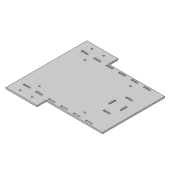
# Autodesk Inventor part: Chassis
Saved by Autodesk Inventor 2017 (Build 210142000, 142)
## iProperties
Created: 2019-06-10
Part Number: Chassis
Material: Generic
Document SubType Name: Modeling
Designer: markg
Density: 1 g/cm^3
Appearance: Default
Author: markg
Autodesk Inventor part; units mm, degrees
ref_plane "YZ Plane" through (0, 0, 0) normal (1, 0, 0) x (0, 1, 0)
ref_plane "XZ Plane" through (0, 0, 0) normal (0, 1, 0) x (-1, 0, 0)
ref_plane "XY Plane" through (0, 0, 0) normal (0, 0, 1) x (1, 0, 0)
sketch "Sketch1" plane through (0, 0, 0) normal (0, 1, 0) x (-1, 0, 0)
  line L0 (-88.9, 63.5) -> (88.9, 63.5)
  line L1 (88.9, 63.5) -> (88.9, -63.5)
  line L2 (88.9, -63.5) -> (-88.9, -63.5)
  line L3 (-88.9, -63.5) -> (-88.9, 63.5)
  line L4 (-88.9, 63.5) -> (88.9, -63.5) construction
  line L5 (88.9, 63.5) -> (-88.9, -63.5) construction
  point P0 (0, 0)
  dimension "d0" = 127
  dimension "d1" = 177.8
  constraints: 12 end point, 2 midpoint, 2 parallel, 1 horizontal, 1 perpendicular
  measures "d0" distance of L0.start L2.end
  measures "d1" distance of L2.end L1.end
extrude "Extrusion1" add sketch "Sketch1" along normal blind 2.921
sketch "Sketch2" plane through (0, 2.921, 0) normal (0, 1, 0) x (1, 0, 0)
  line L0 (-60.325, -50) -> (39.675, -50) construction
  line L1 (39.675, -50) -> (39.675, 50) construction
  line L2 (39.675, 50) -> (-60.325, 50) construction
  line L3 (-60.325, 50) -> (-60.325, -50) construction
  circle A0 centre (36.119, -46.444) radius 1.5875
  circle A1 centre (-56.769, -46.444) radius 1.5875
  circle A2 centre (-56.769, 46.444) radius 1.5875
  circle A3 centre (36.119, 46.444) radius 1.5875
  point P0 (0, 0)
  dimension "d8" = 100
  dimension "d9" = 100
  dimension "d10" = 50
  dimension "d11" = 60.325
  dimension "d12" = 3.175
  dimension "d13" = 3.175
  dimension "d14" = 3.175
  dimension "d15" = 3.175
  dimension "d16" = 3.556
  dimension "d17" = 3.556
  dimension "d18" = 3.556
  dimension "d19" = 3.556
  dimension "d20" = 3.556
  dimension "d21" = 3.556
  dimension "d22" = 3.556
  dimension "d23" = 3.556
  constraints: 8 end point, 4 centre point, 2 parallel, 1 horizontal, 1 perpendicular
  measures "d8" distance of L2.end L1.end
  measures "d9" distance of L1.end L0.end
  measures "d10" distance from line of point (0, 0) L0
  measures "d11" distance from line of L3 point (0, 0)
  measures "d12" diameter of A0
  measures "d13" diameter of A1
  measures "d14" diameter of A2
  measures "d15" diameter of A3
  measures "d16" distance from line of L1 A0.centre
  measures "d17" distance from line of A0.centre L0
  measures "d18" distance from line of A3.centre L1
  measures "d19" distance from line of L2 A3.centre
  measures "d20" distance from line of L2 A2.centre
  measures "d21" distance from line of L3 A2.centre
  measures "d22" distance from line of A1.centre L0
  measures "d23" distance from line of L3 A1.centre
extrude "Extrusion2" cut sketch "Sketch2" against normal blind 25.4
sketch "Sketch4" plane through (0, 2.921, 0) normal (0, 1, 0) x (1, 0, 0)
  line L0 (-76.2, -60.579) -> (-63.5, -60.579)
  line L1 (-63.5, -60.579) -> (-63.5, -57.785)
  line L2 (-63.5, -57.785) -> (-76.2, -57.785)
  line L3 (-76.2, -57.785) -> (-76.2, -60.579)
  line L4 (-76.2, 60.579) -> (-63.5, 60.579)
  line L5 (-63.5, 60.579) -> (-63.5, 57.785)
  line L6 (-63.5, 57.785) -> (-76.2, 57.785)
  line L7 (-76.2, 57.785) -> (-76.2, 60.579)
  line L8 (-88.9, -63.5) -> (88.9, -63.5) projected
  line L9 (-88.9, 63.5) -> (-88.9, -63.5) projected
  line L10 (88.9, 63.5) -> (-88.9, 63.5) projected
  line L11 (-50.8, -60.579) -> (-38.1, -60.579)
  line L12 (-38.1, -60.579) -> (-38.1, -57.785)
  line L13 (-38.1, -57.785) -> (-50.8, -57.785)
  line L14 (-50.8, -57.785) -> (-50.8, -60.579)
  line L15 (-50.8, 60.579) -> (-38.1, 60.579)
  line L16 (-38.1, 60.579) -> (-38.1, 57.785)
  line L17 (-38.1, 57.785) -> (-50.8, 57.785)
  line L18 (-50.8, 57.785) -> (-50.8, 60.579)
  line L19 (-25.4, -60.579) -> (-12.7, -60.579)
  line L20 (-12.7, -60.579) -> (-12.7, -57.785)
  line L21 (-12.7, -57.785) -> (-25.4, -57.785)
  line L22 (-25.4, -57.785) -> (-25.4, -60.579)
  line L23 (-25.4, 60.579) -> (-12.7, 60.579)
  line L24 (-12.7, 60.579) -> (-12.7, 57.785)
  line L25 (-12.7, 57.785) -> (-25.4, 57.785)
  line L26 (-25.4, 57.785) -> (-25.4, 60.579)
  line L27 (0, -60.579) -> (12.7, -60.579)
  line L28 (12.7, -60.579) -> (12.7, -57.785)
  line L29 (12.7, -57.785) -> (0, -57.785)
  line L30 (0, -57.785) -> (0, -60.579)
  line L31 (0, 60.579) -> (12.7, 60.579)
  line L32 (12.7, 60.579) -> (12.7, 57.785)
  line L33 (12.7, 57.785) -> (0, 57.785)
  line L34 (0, 57.785) -> (0, 60.579)
  line L35 (25.4, -60.579) -> (38.1, -60.579)
  line L36 (38.1, -60.579) -> (38.1, -57.785)
  line L37 (38.1, -57.785) -> (25.4, -57.785)
  line L38 (25.4, -57.785) -> (25.4, -60.579)
  line L39 (25.4, 60.579) -> (38.1, 60.579)
  line L40 (38.1, 60.579) -> (38.1, 57.785)
  line L41 (38.1, 57.785) -> (25.4, 57.785)
  line L42 (25.4, 57.785) -> (25.4, 60.579)
  line L43 (50.8, -60.579) -> (63.5, -60.579)
  line L44 (63.5, -60.579) -> (63.5, -57.785)
  line L45 (63.5, -57.785) -> (50.8, -57.785)
  line L46 (50.8, -57.785) -> (50.8, -60.579)
  line L47 (50.8, 60.579) -> (63.5, 60.579)
  line L48 (63.5, 60.579) -> (63.5, 57.785)
  line L49 (63.5, 57.785) -> (50.8, 57.785)
  line L50 (50.8, 57.785) -> (50.8, 60.579)
  point P0 (0, 0)
  point P1 (0, -57.15)
  point P2 (0, 57.15)
  dimension "d26" = 2.794
  dimension "d27" = 2.794
  dimension "d28" = 2.921
  dimension "d29" = 12.7
  dimension "d30" = 12.7
  dimension "d31" = 12.7
  dimension "d32" = 2.921
  dimension "d33" = 12.7
  dimension "d36" = 25.4
  constraints: 96 end point, 4 parallel, 3 horizontal, 2 perpendicular, 1 collinear, 81 other
  measures "d26" distance of L2.end L0.start
  measures "d27" distance of L6.end L4.start
  measures "d29" distance of L1.end L2.end
  measures "d30" distance between parallel lines of L9 L3
  measures "d31" distance of L5.end L6.end
  measures "d33" distance between parallel lines of L9 L7
  measures "d36" distance of L0.start L11.start
extrude "Extrusion3" cut sketch "Sketch4" against normal blind 25.4
sketch "Sketch5" plane through (0, 2.921, 0) normal (0, 1, 0) x (1, 0, 0)
  line L0 (-88.9, 63.5) -> (-25.4, 63.5)
  line L1 (-25.4, 63.5) -> (-25.4, 82.55)
  line L2 (-25.4, 82.55) -> (-88.9, 82.55)
  line L3 (-88.9, 82.55) -> (-88.9, 63.5)
  line L4 (-88.9, -63.5) -> (88.9, -63.5) projected
  line L5 (-88.9, -63.5) -> (-25.4, -63.5)
  line L6 (-25.4, -63.5) -> (-25.4, -82.55)
  line L7 (-25.4, -82.55) -> (-88.9, -82.55)
  line L8 (-88.9, -82.55) -> (-88.9, -63.5)
  line L9 (88.9, 63.5) -> (-88.9, 63.5) projected
  line L10 (-88.9, 63.5) -> (-88.9, -63.5) projected
  point P0 (0, 0)
  point P1 (0, -57.15)
  point P2 (0, 57.15)
  point P3 (88.9, -63.5)
  dimension "d43" = 63.5
  dimension "d44" = 19.05
  dimension "d45" = 63.5
  dimension "d46" = 19.05
  dimension "d47" = 0
  dimension "d64" = 0
  constraints: 16 end point, 4 parallel, 2 horizontal, 2 perpendicular, 2 other
  measures "d43" distance of L6.end L7.end
  measures "d44" distance of L7.end L5.start
  measures "d45" distance of L1.end L2.end
  measures "d46" distance of L2.end L0.start
  measures "d47" vertical extent of L0
  measures "d64" distance between parallel lines of L10 L3
extrude "Extrusion4" add sketch "Sketch5" against normal blind 2.921
sketch "Sketch6" plane through (0, 2.921, 0) normal (0, 1, 0) x (1, 0, 0)
  circle A0 centre (-69.215, 73.025) radius 1.5875
  circle A1 centre (-69.215, -73.025) radius 1.5875
  circle A2 centre (-45.085, -73.025) radius 1.5875
  circle A3 centre (-45.085, 73.025) radius 1.5875
  line L0 (-25.4, 82.55) -> (-88.9, 82.55) projected
  line L1 (-25.4, -82.55) -> (-88.9, -82.55) projected
  line L2 (-88.9, 82.55) -> (-88.9, -82.55) projected
  point P0 (0, 0)
  dimension "d50" = 3.175
  dimension "d51" = 9.525
  dimension "d52" = 9.525
  dimension "d53" = 24.13
  dimension "d54" = 24.13
  dimension "d55" = 9.525
  dimension "d56" = 9.525
  dimension "d57" = 3.175
  dimension "d58" = 3.175
  dimension "d59" = 3.175
  dimension "d61" = 19.685
  dimension "d65" = 19.685
  constraints: 4 centre point
  measures "d50" diameter of A0
  measures "d51" distance from line of L0 A0.centre
  measures "d52" distance from line of A3.centre L0
  measures "d53" distance of A3.centre A0.centre
  measures "d54" distance of A2.centre A1.centre
  measures "d55" distance from line of L1 A2.centre
  measures "d56" distance from line of L1 A1.centre
  measures "d57" diameter of A3
  measures "d58" diameter of A2
  measures "d59" diameter of A1
  measures "d61" distance from line of A1.centre L2
  measures "d65" distance from line of L2 A0.centre
extrude "Extrusion5" cut sketch "Sketch6" against normal blind 2.921
sketch "Sketch7" plane through (0, 2.921, 0) normal (0, 1, 0) x (1, 0, 0)
  line L0 (50.8, 24.003) -> (63.5, 24.003)
  line L1 (63.5, 24.003) -> (63.5, 21.209)
  line L2 (63.5, 21.209) -> (50.8, 21.209)
  line L3 (50.8, 21.209) -> (50.8, 24.003)
  line L4 (50.8, -21.971) -> (63.5, -21.971)
  line L5 (63.5, -21.971) -> (63.5, -24.765)
  line L6 (63.5, -24.765) -> (50.8, -24.765)
  line L7 (50.8, -24.765) -> (50.8, -21.971)
  line L8 (44.196, 6.35) -> (46.99, 6.35)
  line L9 (46.99, 6.35) -> (46.99, -6.35)
  line L10 (46.99, -6.35) -> (44.196, -6.35)
  line L11 (44.196, -6.35) -> (44.196, 6.35)
  line L12 (67.31, 6.35) -> (70.104, 6.35)
  line L13 (70.104, 6.35) -> (70.104, -6.35)
  line L14 (70.104, -6.35) -> (67.31, -6.35)
  line L15 (67.31, -6.35) -> (67.31, 6.35)
  point P0 (0, 0)
  dimension "d66" = 43.18
  dimension "d67" = 12.7
  dimension "d68" = 21.209
  dimension "d69" = 2.794
  dimension "d70" = 2.794
  dimension "d71" = 50.8
  dimension "d72" = 12.7
  dimension "d73" = 6.35
  dimension "d74" = 20.32
  dimension "d75" = 2.794
  dimension "d76" = 2.794
  dimension "d77" = 3.81
  constraints: 32 end point, 8 parallel, 4 horizontal, 4 perpendicular, 4 point on line
  measures "d66" distance between parallel lines of L4 L2
  measures "d67" distance of L5.end L6.end
  measures "d68" distance from line of L2 point (0, 0)
  measures "d69" distance of L0.end L1.end
  measures "d70" distance of L4.end L5.end
  measures "d71" distance from line of point (0, 0) L3
  measures "d72" distance of L10.end L8.start
  measures "d73" distance from line of point (0, 0) L10
  measures "d74" distance between parallel lines of L9 L15
  measures "d75" distance of L8.start L8.end
  measures "d76" distance of L12.start L12.end
  measures "d77" distance between parallel lines of L7 L9
extrude "Extrusion6" cut sketch "Sketch7" against normal blind 2.921
body "Solid1"
